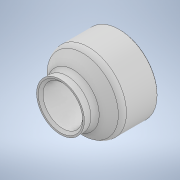
# Autodesk Inventor part: CNC_VacuumCleaner_Adapter
Saved by Autodesk Inventor 2021 (Build 250183000, 183)
## iProperties
Created: 2020-07-24
Part Number: CNC_VacuumCleaner_Adapter
Material: Generic
Document SubType Name: Modeling
Designer: CASE-SMALL2
Density: 1 g/cm^3
Appearance: Default
Author: CASE-SMALL2
## iProperties of the stored document _3DPrint.ipt
Created: 2020-07-24
Part Number: _3DPrint
Material: Generic
Document SubType Name: Modeling
Designer: CASE-SMALL2
Density: 1 g/cm^3
Appearance: Default
Author: CASE-SMALL2
Autodesk Inventor part; units mm, degrees
ref_plane "YZ Plane" through (0, 0, 0) normal (1, 0, 0) x (0, 1, 0)
ref_plane "XZ Plane" through (0, 0, 0) normal (0, 1, 0) x (-1, 0, 0)
sketch "Sketch2" plane through (0, 0, 0) normal (0, 1, 0) x (-1, 0, 0)
  line L0 (-45, 0) -> (7.5, 0) projected
  line L1 (0, -11.9711) -> (0, 71.8268) projected
  line L2 (-37.5, 0) -> (-37.5, 34)
  line L3 (-23.2693, 48.2307) -> (-23.6182, 59.8557)
  line L4 (-19.5, 55.9775) -> (-18, 6)
  line L5 (-19.5, 55.9775) -> (-23.6182, 59.8557)
  line L6 (-33.5, 0) -> (-37.5, 0)
  line L7 (-37.5, 34) -> (-23.2693, 48.2307)
  line L8 (-18, 6) -> (-24, 0)
  line L9 (-33.5, 0) -> (-24, 0)
  point P0 (0, 0)
  dimension "d4" = 4
  dimension "d7" = 34
  dimension "d8" = 37.5
  dimension "d9" = 18
  dimension "d10" = 50
  dimension "d11" = 135
  dimension "d15" = 19.5
  dimension "d25" = 24
  dimension "d26" = 45
  dimension "d27" = 135
  constraints: 16 end point, 3 point on line, 1 collinear, 1 parallel, 1 vertical
  measures "d4" distance between parallel lines of L3 L4
  measures "d7" distance of L2.start L2.end
  measures "d8" distance between parallel lines of L1 L2
  measures "d9" distance from line of L1 L4.end
  measures "d10" distance of L4.start L4.end
  measures "d11" angle of L5 L4
  measures "d15" distance from line of L1 L4.start
  measures "d25" distance from line of L1 L8.end
  measures "d26" angle of L0 L8
  measures "d27" angle of L2 L7
revolve "Revolution1" add sketch "Sketch2" angle 360 about axis through (0, 0, -10) along (0, 0, 1)
fillet "Fillet1" radius 8 2 edges at (-23.2693, 0, 48.2307) (-37.5, 0, 34)
ref_plane "Work Plane1" through (0, 0, 60.25) normal (0, 0, 1) x (1, 0, 0)
sketch "Sketch3" plane through (0, 0, 60.25) normal (0, 0, 1) x (1, 0, 0)
  circle A0 centre (0, 0) radius 31.1812
  constraints: 1 centre point, 1 coincident
extrude "Extrusion2" cut sketch "Sketch3" against normal blind 2
chamfer "Chamfer1" distance 0.5 angle 45 1 edges at (-37.5, 0, 0)
fillet "Fillet2" radius 8 1 edges at (-18, 0, 6)
body "Solid2"
